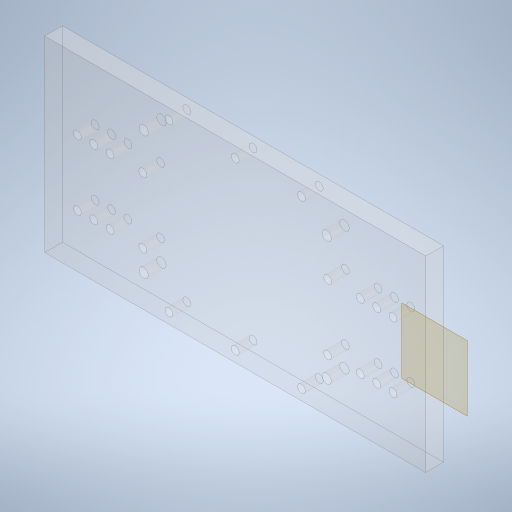
# Autodesk Inventor part: _body_3
Saved by Autodesk Inventor 2024.3 (Build 283343000, 343)
## iProperties
Created: 2024-09-08
Part Number: _body_3
Material: PMMA 플라스틱
Document SubType Name: Modeling
Designer: gretc
Density: 1.188 g/cm^3
Appearance: 폴리카보네이트 - 선명
Mass: 56.5129 g
Surface Area: 195.146 cm^2
Volume: 47.5698 cm^3
Author: gretc
Autodesk Inventor part; units mm, degrees
ref_plane "YZ Plane" through (0, 0, 0) normal (1, 0, 0) x (0, 1, 0)
ref_plane "XZ Plane" through (0, 0, 0) normal (0, 1, 0) x (-1, 0, 0)
ref_plane "XY Plane" through (0, 0, 0) normal (0, 0, 1) x (1, 0, 0)
ref_plane "작업 평면2" through (0, 0, 0) normal (0, 0, 1) x (1, 0, 0)
sketch "스케치1" plane through (0, 0, 0) normal (0, 0, 1) x (1, 0, 0)
  circle A0 centre (-30, -10.6625) radius 1.35 projected
  circle A1 centre (-8, 11.3375) radius 1.35 projected
  circle A2 centre (-19, -10.6625) radius 1.35 projected
  circle A3 centre (-30, 11.3375) radius 1.35 projected
  circle A4 centre (-19, 11.3375) radius 1.35 projected
  circle A5 centre (-8, -10.6625) radius 1.35 projected
  line L0 (3, -32.6625) -> (3, 34.6625) projected
  line L1 (3, 34.6625) -> (-41, 34.6625) projected
  line L2 (-41, -32.6625) -> (-41, 34.6625) projected
  line L3 (3, -32.6625) -> (-41, -32.6625) projected
  circle A6 centre (-92.2, -10.6625) radius 1.35 projected
  circle A7 centre (-114.2, 11.3375) radius 1.35 projected
  circle A8 centre (-103.2, -10.6625) radius 1.35 projected
  circle A9 centre (-92.2, 11.3375) radius 1.35 projected
  circle A10 centre (-103.2, 11.3375) radius 1.35 projected
  circle A11 centre (-114.2, -10.6625) radius 1.35 projected
  line L4 (-125.2, -32.6625) -> (-125.2, 34.6625) projected
  line L5 (-125.2, -32.6625) -> (-81.2, -32.6625) projected
  line L6 (-81.2, -32.6625) -> (-81.2, 34.6625) projected
  line L7 (-125.2, 34.6625) -> (-81.2, 34.6625) projected
  line L8 (3, -28.4172) -> (3, 34.6625)
  line L9 (3, 34.6625) -> (-125.2, 34.6625)
  line L10 (-125.2, 34.6625) -> (-125.2, -28.4172)
  line L11 (-125.2, -28.4172) -> (3, -28.4172)
  point P0 (0, 0)
  point P1 (-41, 34.6625)
  point P2 (-125.2, -28.4172)
  constraints: 8 end point, 2 parallel, 2 perpendicular, 1 point on line
extrude "돌출1" add sketch "스케치1" along normal blind 6 contours L11 L2 L1 L0 | L11 L6 L9 L2 | L11 L4 L7 L6
sketch "스케치2" plane through (0, 0, 6) normal (0, 0, 1) x (1, 0, 0)
  circle A0 centre (-91.9, 23.9225) radius 1.6 projected
  circle A1 centre (-30.3, 23.9225) radius 1.6 projected
  circle A2 centre (-91.9, -17.6775) radius 1.6 projected
  circle A3 centre (-30.3, -17.6775) radius 1.6 projected
  line L0 (-26.1, 28.1225) -> (-96.1, 28.1225) projected
  line L1 (-96.1, 28.1225) -> (-96.1, -21.8775) projected
  line L2 (-96.1, -21.8775) -> (-26.1, -21.8775) projected
  line L3 (-26.1, -21.8775) -> (-26.1, 28.1225) projected
  line L4 (-76.5416, 6.5834) -> (-75.7309, 6.5834) projected
  line L5 (-75.7309, 6.5834) -> (-75.7309, 1.2051) projected
  line L6 (-75.7309, 1.2051) -> (-73.6844, 1.2051) projected
  line L7 (-73.6844, 1.2051) -> (-73.6844, 0.4834) projected
  line L8 (-73.6844, 0.4834) -> (-78.5882, 0.4834) projected
  line L9 (-78.5882, 0.4834) -> (-78.5882, 1.2051) projected
  line L10 (-78.5882, 1.2051) -> (-76.5416, 1.2051) projected
  line L11 (-76.5416, 1.2051) -> (-76.5416, 6.5834) projected
  spline S0 degree 2 poles (-69.4332, 6.1484) (-69.1416, 6.4351) (-68.3704, 6.7119) (-67.8069, 6.7119) knots 0 0 0 1 2 2 2 projected
  spline S1 degree 2 poles (-67.8069, 6.7119) (-67.2681, 6.7119) (-66.4672, 6.4302) (-66.1855, 6.1484) knots 0 0 0 1 2 2 2 projected
  spline S2 degree 2 poles (-66.1855, 6.1484) (-65.8642, 5.832) (-65.6022, 4.9422) (-65.6022, 4.2897) knots 0 0 0 1 2 2 2 projected
  line L12 (-65.6022, 4.2897) -> (-65.6022, 0.4834) projected
  line L13 (-65.6022, 0.4834) -> (-66.4129, 0.4834) projected
  line L14 (-66.4129, 0.4834) -> (-66.4129, 4.2897) projected
  spline S3 degree 2 poles (-66.4129, 4.2897) (-66.4129, 4.7149) (-66.5216, 5.2883) (-66.6749, 5.5206) knots 0 0 0 1 2 2 2 projected
  spline S4 degree 2 poles (-66.6749, 5.5206) (-66.838, 5.7678) (-67.4015, 6.0199) (-67.8069, 6.0199) knots 0 0 0 1 2 2 2 projected
  spline S5 degree 2 poles (-67.8069, 6.0199) (-68.1875, 6.0199) (-68.7807, 5.7678) (-68.9438, 5.5206) knots 0 0 0 1 2 2 2 projected
  spline S6 degree 2 poles (-68.9438, 5.5206) (-69.0971, 5.2883) (-69.2058, 4.7198) (-69.2058, 4.3095) knots 0 0 0 1 2 2 2 projected
  line L15 (-69.2058, 4.3095) -> (-69.2058, 0.4834) projected
  line L16 (-69.2058, 0.4834) -> (-70.0165, 0.4834) projected
  line L17 (-70.0165, 0.4834) -> (-70.0165, 4.2897) projected
  spline S7 degree 2 poles (-70.0165, 4.2897) (-70.0165, 4.9274) (-69.7595, 5.837) (-69.4332, 6.1484) knots 0 0 0 1 2 2 2 projected
  line L18 (-54.4304, 5.9606) -> (-54.4304, 6.5834) projected
  line L19 (-54.4304, 6.5834) -> (-52.0675, 6.5834) projected
  line L20 (-52.0675, 6.5834) -> (-52.0675, 5.9606) projected
  line L21 (-52.0675, 5.9606) -> (-52.8436, 5.9606) projected
  line L22 (-52.8436, 5.9606) -> (-52.8436, 1.1063) projected
  line L23 (-52.8436, 1.1063) -> (-52.0675, 1.1063) projected
  line L24 (-52.0675, 1.1063) -> (-52.0675, 0.4834) projected
  line L25 (-52.0675, 0.4834) -> (-54.4304, 0.4834) projected
  line L26 (-54.4304, 0.4834) -> (-54.4304, 1.1063) projected
  line L27 (-54.4304, 1.1063) -> (-53.6543, 1.1063) projected
  line L28 (-53.6543, 1.1063) -> (-53.6543, 5.9606) projected
  line L29 (-53.6543, 5.9606) -> (-54.4304, 5.9606) projected
  spline S8 degree 2 poles (-50.7377, 6.5142) (-50.4708, 6.6032) (-50.016, 6.6922) (-49.6502, 6.6922) knots 0 0 0 1 2 2 2 projected
  spline S9 degree 2 poles (-49.6502, 6.6922) (-49.057, 6.6922) (-48.0536, 6.2918) (-47.6877, 5.8914) knots 0 0 0 1 2 2 2 projected
  spline S10 degree 2 poles (-47.6877, 5.8914) (-47.3219, 5.4959) (-46.9215, 4.3095) (-46.9215, 3.5384) knots 0 0 0 1 2 2 2 projected
  spline S11 degree 2 poles (-46.9215, 3.5384) (-46.9215, 2.7721) (-47.3121, 1.6352) (-47.6828, 1.215) knots 0 0 0 1 2 2 2 projected
  spline S12 degree 2 poles (-47.6828, 1.215) (-48.0486, 0.8047) (-49.0471, 0.3747) (-49.6651, 0.3747) knots 0 0 0 1 2 2 2 projected
  spline S13 degree 2 poles (-49.6651, 0.3747) (-49.9715, 0.3747) (-50.5104, 0.4636) (-50.7377, 0.5328) knots 0 0 0 1 2 2 2 projected
  spline S14 degree 2 poles (-50.7377, 0.5328) (-50.9355, 0.5971) (-51.3458, 0.78) (-51.5484, 0.8888) knots 0 0 0 1 2 2 2 projected
  line L30 (-51.5484, 0.8888) -> (-51.5484, 1.8675) projected
  line L31 (-51.5484, 1.8675) -> (-51.4842, 1.8675) projected
  spline S15 degree 2 poles (-51.4842, 1.8675) (-51.3754, 1.7687) (-51.0393, 1.4918) (-50.7971, 1.3584) knots 0 0 0 1 2 2 2 projected
  spline S16 degree 2 poles (-50.7971, 1.3584) (-50.5647, 1.2298) (-50.016, 1.0667) (-49.6601, 1.0667) knots 0 0 0 1 2 2 2 projected
  spline S17 degree 2 poles (-49.6601, 1.0667) (-49.2696, 1.0667) (-48.5726, 1.388) (-48.3106, 1.6945) knots 0 0 0 1 2 2 2 projected
  spline S18 degree 2 poles (-48.3106, 1.6945) (-48.0536, 2.0059) (-47.7668, 2.9501) (-47.7668, 3.5384) knots 0 0 0 1 2 2 2 projected
  spline S19 degree 2 poles (-47.7668, 3.5384) (-47.7668, 4.1662) (-48.0684, 5.0708) (-48.3304, 5.3822) knots 0 0 0 1 2 2 2 projected
  spline S20 degree 2 poles (-48.3304, 5.3822) (-48.5874, 5.6837) (-49.2745, 5.9902) (-49.6601, 5.9902) knots 0 0 0 1 2 2 2 projected
  spline S21 degree 2 poles (-49.6601, 5.9902) (-50.0111, 5.9902) (-50.6092, 5.8172) (-50.8416, 5.6887) knots 0 0 0 1 2 2 2 projected
  spline S22 degree 2 poles (-50.8416, 5.6887) (-51.064, 5.5602) (-51.3952, 5.2932) (-51.4891, 5.1993) knots 0 0 0 1 2 2 2 projected
  line L32 (-51.4891, 5.1993) -> (-51.5484, 5.1993) projected
  line L33 (-51.5484, 5.1993) -> (-51.5484, 6.1682) projected
  spline S23 degree 2 poles (-51.5484, 6.1682) (-51.3458, 6.2621) (-50.9899, 6.4351) (-50.7377, 6.5142) knots 0 0 0 1 2 2 2 projected
  line L34 (-57.9846, 3.9289) -> (-60.1547, 6.5834) projected
  line L35 (-60.1547, 6.5834) -> (-59.1018, 6.5834) projected
  line L36 (-59.1018, 6.5834) -> (-57.1739, 4.1563) projected
  line L37 (-57.1739, 4.1563) -> (-56.2446, 4.1563) projected
  line L38 (-56.2446, 4.1563) -> (-56.2446, 6.5834) projected
  line L39 (-56.2446, 6.5834) -> (-55.4339, 6.5834) projected
  line L40 (-55.4339, 6.5834) -> (-55.4339, 0.4834) projected
  line L41 (-55.4339, 0.4834) -> (-57.0058, 0.4834) projected
  spline S24 degree 2 poles (-57.0058, 0.4834) (-57.5298, 0.4834) (-58.2367, 0.5971) (-58.558, 0.8047) knots 0 0 0 1 2 2 2 projected
  spline S25 degree 2 poles (-58.558, 0.8047) (-58.8793, 1.0123) (-59.2501, 1.6599) (-59.2501, 2.1394) knots 0 0 0 1 2 2 2 projected
  spline S26 degree 2 poles (-59.2501, 2.1394) (-59.2501, 2.8068) (-58.5679, 3.7114) (-57.9846, 3.9289) knots 0 0 0 1 2 2 2 projected
  spline S27 degree 2 poles (-64.1093, 6.5142) (-63.8424, 6.6032) (-63.3876, 6.6922) (-63.0218, 6.6922) knots 0 0 0 1 2 2 2 projected
  spline S28 degree 2 poles (-63.0218, 6.6922) (-62.4286, 6.6922) (-61.4251, 6.2918) (-61.0593, 5.8914) knots 0 0 0 1 2 2 2 projected
  spline S29 degree 2 poles (-61.0593, 5.8914) (-60.6935, 5.4959) (-60.2931, 4.3095) (-60.2931, 3.5384) knots 0 0 0 1 2 2 2 projected
  spline S30 degree 2 poles (-60.2931, 3.5384) (-60.2931, 2.7721) (-60.6836, 1.6352) (-61.0544, 1.215) knots 0 0 0 1 2 2 2 projected
  spline S31 degree 2 poles (-61.0544, 1.215) (-61.4202, 0.8047) (-62.4187, 0.3747) (-63.0366, 0.3747) knots 0 0 0 1 2 2 2 projected
  spline S32 degree 2 poles (-63.0366, 0.3747) (-63.3431, 0.3747) (-63.8819, 0.4636) (-64.1093, 0.5328) knots 0 0 0 1 2 2 2 projected
  spline S33 degree 2 poles (-64.1093, 0.5328) (-64.307, 0.5971) (-64.7173, 0.78) (-64.92, 0.8888) knots 0 0 0 1 2 2 2 projected
  line L42 (-64.92, 0.8888) -> (-64.92, 1.8675) projected
  line L43 (-64.92, 1.8675) -> (-64.8557, 1.8675) projected
  spline S34 degree 2 poles (-64.8557, 1.8675) (-64.747, 1.7687) (-64.4108, 1.4918) (-64.1686, 1.3584) knots 0 0 0 1 2 2 2 projected
  spline S35 degree 2 poles (-64.1686, 1.3584) (-63.9363, 1.2298) (-63.3876, 1.0667) (-63.0317, 1.0667) knots 0 0 0 1 2 2 2 projected
  spline S36 degree 2 poles (-63.0317, 1.0667) (-62.6412, 1.0667) (-61.9442, 1.388) (-61.6822, 1.6945) knots 0 0 0 1 2 2 2 projected
  spline S37 degree 2 poles (-61.6822, 1.6945) (-61.4251, 2.0059) (-61.1384, 2.9501) (-61.1384, 3.5384) knots 0 0 0 1 2 2 2 projected
  spline S38 degree 2 poles (-61.1384, 3.5384) (-61.1384, 4.1662) (-61.4399, 5.0708) (-61.7019, 5.3822) knots 0 0 0 1 2 2 2 projected
  spline S39 degree 2 poles (-61.7019, 5.3822) (-61.959, 5.6837) (-62.6461, 5.9902) (-63.0317, 5.9902) knots 0 0 0 1 2 2 2 projected
  spline S40 degree 2 poles (-63.0317, 5.9902) (-63.3826, 5.9902) (-63.9808, 5.8172) (-64.2131, 5.6887) knots 0 0 0 1 2 2 2 projected
  spline S41 degree 2 poles (-64.2131, 5.6887) (-64.4356, 5.5602) (-64.7668, 5.2932) (-64.8607, 5.1993) knots 0 0 0 1 2 2 2 projected
  line L44 (-64.8607, 5.1993) -> (-64.92, 5.1993) projected
  line L45 (-64.92, 5.1993) -> (-64.92, 6.1682) projected
  spline S42 degree 2 poles (-64.92, 6.1682) (-64.7173, 6.2621) (-64.3614, 6.4351) (-64.1093, 6.5142) knots 0 0 0 1 2 2 2 projected
  line L46 (-73.3038, 5.9606) -> (-73.3038, 6.5834) projected
  line L47 (-73.3038, 6.5834) -> (-70.9409, 6.5834) projected
  line L48 (-70.9409, 6.5834) -> (-70.9409, 5.9606) projected
  line L49 (-70.9409, 5.9606) -> (-71.717, 5.9606) projected
  line L50 (-71.717, 5.9606) -> (-71.717, 1.1063) projected
  line L51 (-71.717, 1.1063) -> (-70.9409, 1.1063) projected
  line L52 (-70.9409, 1.1063) -> (-70.9409, 0.4834) projected
  line L53 (-70.9409, 0.4834) -> (-73.3038, 0.4834) projected
  line L54 (-73.3038, 0.4834) -> (-73.3038, 1.1063) projected
  line L55 (-73.3038, 1.1063) -> (-72.5277, 1.1063) projected
  line L56 (-72.5277, 1.1063) -> (-72.5277, 5.9606) projected
  line L57 (-72.5277, 5.9606) -> (-73.3038, 5.9606) projected
  line L58 (-96.1, 28.1225) -> (-26.1, -21.8775)
  line L59 (-96.1, -21.8775) -> (-26.1, 28.1225)
  line L60 (-20.1, -27.8775) -> (-102.1, -27.8775)
  line L61 (-102.1, -21.996) -> (-102.1, 28.2411)
  line L62 (-102.1, 34.1225) -> (-20.1, 34.1225)
  line L63 (-20.1, 28.2411) -> (-20.1, -21.996)
  line L64 (-20.1, -27.8775) -> (-102.1, 34.1225) construction
  line L65 (-102.1, -27.8775) -> (-20.1, 34.1225) construction
  circle A4 centre (-114.2, 11.3375) radius 1.35 projected
  circle A5 centre (-103.2, 11.3375) radius 1.35 projected
  line L66 (-114.2, 11.3375) -> (-103.2, 11.3375)
  line L67 (-103.2, 11.3375) -> (-108.7, 11.3375)
  line L68 (-108.7, 11.3375) -> (-105.7, 11.3375)
  line L69 (-108.7, 11.3375) -> (-111.7, 11.3375)
  line L70 (-111.7, 11.3375) -> (-105.7, 11.3375)
  line L71 (-105.7, -28.4172) -> (-111.7, -28.4172)
  line L72 (-111.7, -27.8775) -> (-111.7, 11.3375)
  line L73 (-111.7, 11.3375) -> (-105.7, 11.3375)
  line L74 (-105.7, 34.6625) -> (-111.7, 34.6625)
  line L75 (-111.7, 34.1225) -> (-111.7, 11.3375)
  line L76 (-102.1, 34.1225) -> (-111.7, 34.1225)
  line L77 (-102.1, -27.8775) -> (-111.7, -27.8775)
  line L78 (-10.5, -27.8775) -> (-111.7, -27.8775)
  line L79 (-111.7, -27.8775) -> (-111.7, 34.1225)
  line L80 (-111.7, 34.1225) -> (-10.5, 34.1225)
  line L81 (-10.5, 34.1225) -> (-10.5, -27.8775)
  line L82 (-10.5, -27.8775) -> (-111.7, 34.1225) construction
  line L83 (-102.1, -21.996) -> (-10.5, 34.1225) construction
  line L84 (-16.5, -21.8775) -> (-105.7, -21.8775)
  line L85 (-105.7, -21.8775) -> (-105.7, 28.1225)
  line L86 (-105.7, 28.1225) -> (-16.5, 28.1225)
  line L87 (-16.5, 28.1225) -> (-16.5, -21.8775)
  line L88 (-16.5, -21.8775) -> (-105.7, 28.1225) construction
  line L89 (-105.7, -21.8775) -> (-16.5, 28.1225) construction
  line L90 (-105.7, 11.3375) -> (-105.7, 28.1225)
  line L91 (-105.7, 11.3375) -> (-105.7, -21.8775)
  line L92 (-105.7, -21.8775) -> (-105.7, -27.8775)
  line L93 (-16.5, -21.8775) -> (-16.5, -27.8775)
  line L94 (-16.5, 28.1225) -> (-16.5, 34.1225)
  line L95 (-105.7, 28.1225) -> (-105.7, 34.1225)
  line L96 (3, -28.4172) -> (3, 34.6625) projected
  line L97 (3, 34.6625) -> (-125.2, 34.6625) projected
  line L98 (-125.2, 34.6625) -> (-125.2, -28.4172) projected
  line L99 (-125.2, -28.4172) -> (3, -28.4172) projected
  circle A6 centre (-114.2, -10.6625) radius 1.35 projected
  circle A7 centre (-92.2, 11.3375) radius 1.35 projected
  circle A8 centre (-114.2, 11.3375) radius 1.35 projected
  circle A9 centre (-92.2, -10.6625) radius 1.35 projected
  circle A10 centre (-103.2, -10.6625) radius 1.35 projected
  circle A11 centre (-103.2, 11.3375) radius 1.35 projected
  circle A12 centre (-30, -10.6625) radius 1.35 projected
  circle A13 centre (-8, 11.3375) radius 1.35 projected
  circle A14 centre (-19, -10.6625) radius 1.35 projected
  circle A15 centre (-30, 11.3375) radius 1.35 projected
  circle A16 centre (-19, 11.3375) radius 1.35 projected
  circle A17 centre (-8, -10.6625) radius 1.35 projected
  line L100 (-114.2, 11.3375) -> (-103.2, 11.3375)
  line L101 (-103.2, 11.3375) -> (-103.2, -10.6625)
  line L102 (-103.2, -10.6625) -> (-114.2, -10.6625)
  line L103 (-114.2, -10.6625) -> (-114.2, 11.3375)
  line L104 (-108.7, 11.3375) -> (-108.7, -10.6625)
  circle A18 centre (-108.7, -10.6625) radius 1.35
  circle A19 centre (-108.7, 11.3375) radius 1.3956
  line L105 (-8, 11.3375) -> (-19, 11.3375)
  line L106 (-19, 11.3375) -> (-19, -10.6625)
  line L107 (-19, -10.6625) -> (-8, -10.6625)
  line L108 (-8, -10.6625) -> (-8, 11.3375)
  line L109 (-13.5, 11.3375) -> (-13.5, -10.6625)
  circle A20 centre (-13.5, 11.3375) radius 1.35
  circle A21 centre (-13.5, -10.6625) radius 1.35
  line L110 (-16.5, 34.1225) -> (-38.8, 34.1225)
  line L111 (-16.5, 34.1225) -> (5.8, 34.1225) construction
  line L112 (-38.8, 34.1225) -> (-61.1, 34.1225)
  line L113 (-61.1, 34.1225) -> (-83.4, 34.1225)
  line L114 (-83.4, 34.1225) -> (-83.4, 28.1225)
  line L115 (-61.1, 34.1225) -> (-61.1, 28.1225)
  line L116 (-38.8, 34.1225) -> (-38.8, 28.1225)
  line L117 (-83.4, 31.1225) -> (-38.8, 31.1225)
  circle A22 centre (-83.4, 31.1225) radius 1.35
  circle A23 centre (-61.1, 31.1225) radius 1.35
  circle A24 centre (-38.8, 31.1225) radius 1.35
  line L118 (-83.4, 31.1225) -> (-83.4, -27.8775)
  line L119 (-61.1, 31.1225) -> (-61.1, -27.8775)
  line L120 (-38.8, 31.1225) -> (-38.8, -27.8775)
  line L121 (-83.4, -27.8775) -> (-83.4, -24.8775)
  line L122 (-83.4, -24.8775) -> (-33.4, -24.8775)
  circle A25 centre (-83.4, -24.8775) radius 1.35
  circle A26 centre (-61.1, -24.8775) radius 1.35
  circle A27 centre (-38.8, -24.8775) radius 1.35
  point P0 (0, 0)
  point P1 (-61.1, 3.1225)
  dimension "d2" = 82
  dimension "d3" = 62
  dimension "d4" = 3
  dimension "d5" = 3
  dimension "d6" = 2.7
  dimension "d7" = 2.7
  dimension "d8" = 2.7
  dimension "d9" = 22.3
  dimension "d10" = 180
  dimension "d11" = 22.3
  dimension "d12" = 22.3
  dimension "d13" = 180
  dimension "d14" = 2.7
  dimension "d15" = 2.7
  dimension "d16" = 2.7
  dimension "d17" = 3
  dimension "d18" = 50
  dimension "d19" = 90
  dimension "d20" = 2.7
  dimension "d21" = 2.7
  dimension "d22" = 2.7
  constraints: 122 end point, 21 point on line, 18 perpendicular, 16 midpoint, 15 parallel, 13 coincident, 10 centre point, 5 horizontal, 4 collinear
  measures "d2" distance of L60.start L60.end
  measures "d3" distance of L60.end L62.start
  measures "d4" distance of L67.end L68.end
  measures "d5" distance of L67.end L69.end
  measures "d6" diameter of A18
  measures "d7" diameter of A20
  measures "d8" diameter of A21
  measures "d9" distance of L94.end L110.end
  measures "d10" angle of L111 L110
  measures "d11" distance of L110.end L112.end
  measures "d12" distance of L112.end L113.end
  measures "d13" angle of L112 L113
  measures "d14" diameter of A22
  measures "d15" diameter of A23
  measures "d16" diameter of A24
  measures "d17" distance of L118.end L121.end
  measures "d18" distance of L121.end L122.end
  measures "d19" angle of L121 L122
  measures "d20" diameter of A25
  measures "d21" diameter of A26
  measures "d22" diameter of A27
extrude "돌출2" cut sketch "스케치2" against normal up to surface (6 mm away) contours A22 L114 | L114 L117 A22 | A23 L117 L115 | L115 L117 A23 | L114 A22 L117 | A25 L122 L118 | L118 A25 | A24 L117 L116 | L116 A24 | L117 A23 L115 | L115 A23 L117 | A26 L122 L119 | L119 L122 A26 | L122 A25 L118 | A19 L104 L66 | L66 A19 | L117 A24 L116 | A27 L122 L120 | L120 L122 A27 | L122 A26 L119 | L119 A26 L122 | A18 L102 | L102 L104 A18 | L104 A19 L66 | L122 A27 L120 | L120 A27 L122 | L102 A18 L104 | A20 L105 | L105 L109 A20 | A21 L109 L107 | L107 A21 | L105 A20 L109 | L109 A21 L107
sketch "스케치3" plane through (0, 0, 6) normal (0, 0, 1) x (1, 0, 0)
  circle A0 centre (-91.9, 23.9225) radius 1.6 projected
  circle A1 centre (-91.9, -17.6775) radius 1.6 projected
  circle A2 centre (-30.3, 23.9225) radius 1.6 projected
  circle A3 centre (-30.3, -17.6775) radius 1.6 projected
  point P0 (0, 0)
extrude "돌출3" cut sketch "스케치3" against normal blind 6
